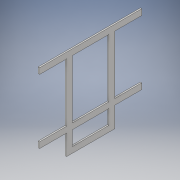
# Autodesk Inventor part: CapBallLiftBacking
Saved by Autodesk Inventor 2017 (Build 210142000, 142)
## iProperties
Created: 2017-06-24
Part Number: CapBallLiftBacking
Material: Generic
Document SubType Name: Modeling
Designer: User
Density: 1 g/cm^3
Appearance: Default
Author: User
Autodesk Inventor part; units mm, degrees
ref_plane "YZ Plane" through (0, 0, 0) normal (1, 0, 0) x (0, 1, 0)
ref_plane "XZ Plane" through (0, 0, 0) normal (0, 1, 0) x (-1, 0, 0)
ref_plane "XY Plane" through (0, 0, 0) normal (0, 0, 1) x (1, 0, 0)
sketch "Sketch1" plane through (0, 0, 0) normal (1, 0, 0) x (0, 1, 0)
  line L0 (0, 0) -> (-114.3, 0)
  line L1 (-114.3, 0) -> (-114.3, -444.5)
  line L2 (-114.3, -444.5) -> (0, -444.5)
  line L3 (-114.3, 0) -> (-25.4, 0)
  line L4 (-25.4, 0) -> (-25.4, -117.6782)
  line L5 (-25.4, -117.6782) -> (-114.3, -117.6782)
  line L6 (-114.3, -117.6782) -> (-114.3, 0)
  line L7 (-114.3, -444.5) -> (-25.4, -444.5)
  line L8 (-25.4, -444.5) -> (-25.4, -326.8218)
  line L9 (-25.4, -326.8218) -> (-114.3, -326.8218)
  line L10 (-114.3, -326.8218) -> (-114.3, -444.5)
  line L11 (-25.4, -143.0782) -> (-88.9, -143.0782)
  line L12 (-88.9, -143.0782) -> (-88.9, -301.4218)
  line L13 (-88.9, -301.4218) -> (-25.4, -301.4218)
  line L14 (-25.4, -301.4218) -> (-25.4, -143.0782)
  line L15 (279.4, -117.6782) -> (279.4, -326.8218)
  line L16 (-114.3, -326.8218) -> (-114.3, -117.6782)
  line L17 (0, -143.0782) -> (254, -143.0782)
  line L18 (254, -143.0782) -> (254, -301.4218)
  line L19 (254, -301.4218) -> (0, -301.4218)
  line L20 (0, -301.4218) -> (0, -143.0782)
  line L21 (0, -117.6782) -> (0, 0)
  line L22 (0, -444.5) -> (0, -326.8218)
  line L23 (0, -301.4218) -> (0, -143.0782)
  line L24 (-114.3, -117.6782) -> (-25.4, -117.6782)
  line L25 (0, -117.6782) -> (254, -117.6782)
  line L26 (254, -326.8218) -> (0, -326.8218)
  line L27 (-25.4, -326.8218) -> (-114.3, -326.8218)
  line L28 (254, -326.8218) -> (254, -444.5)
  line L29 (254, -444.5) -> (279.4, -444.5)
  line L30 (279.4, -444.5) -> (279.4, -326.8218)
  line L31 (254, -117.6782) -> (254, 0)
  line L32 (254, 0) -> (279.4, 0)
  line L33 (279.4, 0) -> (279.4, -117.6782)
  dimension "d0" = 114.3
  dimension "d1" = 444.5
  dimension "d2" = 88.9
  dimension "d3" = 209.1436
  dimension "d4" = 117.6782
  dimension "d9" = 63.5
  dimension "d10" = 158.3436
  dimension "d11" = 25.4
  dimension "d12" = 25.4
  dimension "d16" = 254
  dimension "d24" = 117.6782
  dimension "d25" = 25.4
  dimension "d26" = 117.6782
  dimension "d27" = 25.4
  dimension "d28" = 393.7
  constraints: 68 end point, 19 parallel, 7 horizontal, 7 perpendicular, 2 point on line
  measures "d0" distance of L2.end L1.end
  measures "d1" distance of L0.end L1.end
  measures "d2" distance of L4.end L5.end
  measures "d3" distance between parallel lines of L9 L5
  measures "d4" distance of L3.end L4.end
  measures "d9" distance of L13.end L12.end
  measures "d10" distance of L12.end L11.end
  measures "d11" distance between parallel lines of L5 L11
  measures "d12" distance between parallel lines of L1 L12
  measures "d16" distance of L18.end L19.end
  measures "d24" distance of L25.end L31.end
  measures "d25" distance of L31.end L32.end
  measures "d26" distance of L26.start L28.end
  measures "d27" distance of L28.end L29.end
  measures "d28" distance between parallel lines of L6 L15
extrude "Extrusion2" add sketch "Sketch1" along normal blind 6.35 contours L21 L25 L31 L32 L33 L15 L30 L29 L28 L26 L22 L2 L8 L9 L1 L5 L4 L0
body "Solid2"
